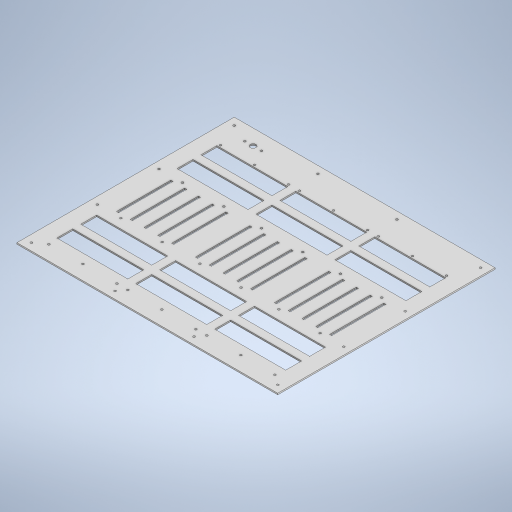
# Autodesk Inventor part: Pannello frontale
Saved by Autodesk Inventor 2023 (Build 270158000, 158)
## iProperties
Created: 2022-05-03
Part Number: Pannello frontale
Material: Generico
Document SubType Name: Sheet Metal
Designer: franc
Density: 1 g/cm^3
Sheet Metal Rule: Default_mm
Appearance: Default
Author: franc
Autodesk Inventor part; units mm, degrees
ref_plane "YZ Plane" through (0, 0, 0) normal (1, 0, 0) x (0, 1, 0)
ref_plane "XZ Plane" through (0, 0, 0) normal (0, 1, 0) x (-1, 0, 0)
ref_plane "XY Plane" through (0, 0, 0) normal (0, 0, 1) x (1, 0, 0)
sketch "Schizzo1" plane through (0, 0, 0) normal (0, 1, 0) x (-1, 0, 0)
  line L0 (270.7569, 212.2832) -> (267.7569, 212.2832)
  line L1 (270.7569, 137.2832) -> (267.7569, 137.2832)
  line L2 (270.7569, 137.2832) -> (270.7569, 212.2832)
  line L3 (267.7569, 137.2832) -> (267.7569, 212.2832)
  line L4 (289.7569, 212.2832) -> (286.7569, 212.2832)
  line L5 (289.7569, 137.2832) -> (286.7569, 137.2832)
  line L6 (289.7569, 137.2832) -> (289.7569, 212.2832)
  line L7 (286.7569, 137.2832) -> (286.7569, 212.2832)
  line L8 (308.7569, 212.2832) -> (305.7569, 212.2832)
  line L9 (308.7569, 137.2832) -> (305.7569, 137.2832)
  line L10 (308.7569, 137.2832) -> (308.7569, 212.2832)
  line L11 (305.7569, 137.2832) -> (305.7569, 212.2832)
  line L12 (327.7569, 212.2832) -> (324.7569, 212.2832)
  line L13 (327.7569, 137.2832) -> (324.7569, 137.2832)
  line L14 (327.7569, 137.2832) -> (327.7569, 212.2832)
  line L15 (324.7569, 137.2832) -> (324.7569, 212.2832)
  line L16 (346.7569, 212.2832) -> (343.7569, 212.2832)
  line L17 (346.7569, 137.2832) -> (343.7569, 137.2832)
  line L18 (346.7569, 137.2832) -> (346.7569, 212.2832)
  line L19 (343.7569, 137.2832) -> (343.7569, 212.2832)
  line L20 (71.7569, 137.2832) -> (68.7569, 137.2832)
  line L21 (71.7569, 137.2832) -> (71.7569, 212.2832)
  line L22 (68.7569, 137.2832) -> (68.7569, 212.2832)
  line L23 (343.7569, 137.2832) -> (346.7569, 137.2832)
  line L24 (90.7569, 137.2832) -> (87.7569, 137.2832)
  line L25 (90.7569, 137.2832) -> (90.7569, 212.2832)
  line L26 (87.7569, 137.2832) -> (87.7569, 212.2832)
  line L27 (109.7569, 212.2832) -> (106.7569, 212.2832)
  line L28 (109.7569, 137.2832) -> (106.7569, 137.2832)
  line L29 (109.7569, 137.2832) -> (109.7569, 212.2832)
  line L30 (106.7569, 137.2832) -> (106.7569, 212.2832)
  line L31 (128.7569, 212.2832) -> (125.7569, 212.2832)
  line L32 (128.7569, 137.2832) -> (125.7569, 137.2832)
  line L33 (128.7569, 137.2832) -> (128.7569, 212.2832)
  line L34 (125.7569, 137.2832) -> (125.7569, 212.2832)
  line L35 (138.2569, 263.2832) -> (40.2569, 263.2832)
  line L36 (90.7569, 212.2832) -> (87.7569, 212.2832)
  line L37 (40.2569, 263.2832) -> (40.2569, 285.2832)
  line L38 (40.2569, 285.2832) -> (138.2569, 285.2832)
  line L39 (138.2569, 285.2832) -> (138.2569, 263.2832)
  line L40 (378.2569, 18.2832) -> (18.2569, 18.2832)
  line L41 (18.2569, 18.2832) -> (18.2569, 318.2832)
  line L42 (18.2569, 318.2832) -> (378.2569, 318.2832)
  line L43 (378.2569, 318.2832) -> (378.2569, 18.2832)
  line L44 (161.7569, 212.2832) -> (158.7569, 212.2832)
  line L45 (161.7569, 137.2832) -> (158.7569, 137.2832)
  line L46 (161.7569, 137.2832) -> (161.7569, 212.2832)
  line L47 (158.7569, 137.2832) -> (158.7569, 212.2832)
  line L48 (180.7569, 212.2832) -> (177.7569, 212.2832)
  line L49 (180.7569, 137.2832) -> (177.7569, 137.2832)
  line L50 (180.7569, 137.2832) -> (180.7569, 212.2832)
  line L51 (177.7569, 137.2832) -> (177.7569, 212.2832)
  line L52 (199.7569, 212.2832) -> (196.7569, 212.2832)
  line L53 (199.7569, 137.2832) -> (196.7569, 137.2832)
  line L54 (199.7569, 137.2832) -> (199.7569, 212.2832)
  line L55 (196.7569, 137.2832) -> (196.7569, 212.2832)
  line L56 (218.7569, 212.2832) -> (215.7569, 212.2832)
  line L57 (218.7569, 137.2832) -> (215.7569, 137.2832)
  line L58 (218.7569, 137.2832) -> (218.7569, 212.2832)
  line L59 (215.7569, 137.2832) -> (215.7569, 212.2832)
  line L60 (237.7569, 212.2832) -> (234.7569, 212.2832)
  line L61 (237.7569, 137.2832) -> (234.7569, 137.2832)
  line L62 (237.7569, 137.2832) -> (237.7569, 212.2832)
  line L63 (234.7569, 137.2832) -> (234.7569, 212.2832)
  line L64 (52.7569, 212.2832) -> (49.7569, 212.2832)
  line L65 (52.7569, 137.2832) -> (49.7569, 137.2832)
  line L66 (52.7569, 137.2832) -> (52.7569, 212.2832)
  line L67 (49.7569, 137.2832) -> (49.7569, 212.2832)
  line L68 (71.7569, 212.2832) -> (68.7569, 212.2832)
  line L69 (149.2569, 263.2832) -> (149.2569, 285.2832)
  line L70 (138.2569, 230.2831) -> (40.2569, 230.2831)
  line L71 (40.2569, 230.2831) -> (40.2569, 252.2831)
  line L72 (40.2569, 252.2831) -> (138.2569, 252.2831)
  line L73 (138.2569, 252.2831) -> (138.2569, 230.2831)
  line L74 (138.2569, 97.2832) -> (40.2569, 97.2832)
  line L75 (40.2569, 97.2832) -> (40.2569, 119.2832)
  line L76 (40.2569, 119.2832) -> (138.2569, 119.2832)
  line L77 (138.2569, 119.2832) -> (138.2569, 97.2832)
  line L78 (138.2569, 64.2832) -> (40.2569, 64.2832)
  line L79 (40.2569, 64.2832) -> (40.2569, 86.2832)
  line L80 (40.2569, 86.2832) -> (138.2569, 86.2832)
  line L81 (138.2569, 86.2832) -> (138.2569, 64.2832)
  line L82 (247.2569, 263.2832) -> (149.2569, 263.2832)
  line L83 (149.2569, 285.2832) -> (247.2569, 285.2832)
  line L84 (247.2569, 285.2832) -> (247.2569, 263.2832)
  line L85 (247.2569, 230.2831) -> (149.2569, 230.2831)
  line L86 (149.2569, 230.2831) -> (149.2569, 252.2831)
  line L87 (149.2569, 252.2831) -> (247.2569, 252.2831)
  line L88 (247.2569, 252.2831) -> (247.2569, 230.2831)
  line L89 (247.2569, 97.2832) -> (149.2569, 97.2832)
  line L90 (149.2569, 97.2832) -> (149.2569, 119.2832)
  line L91 (149.2569, 119.2832) -> (247.2569, 119.2832)
  line L92 (247.2569, 119.2832) -> (247.2569, 97.2832)
  line L93 (247.2569, 64.2832) -> (149.2569, 64.2832)
  line L94 (149.2569, 64.2832) -> (149.2569, 86.2832)
  line L95 (149.2569, 86.2832) -> (247.2569, 86.2832)
  line L96 (247.2569, 86.2832) -> (247.2569, 64.2832)
  line L97 (356.2569, 263.2832) -> (258.2569, 263.2832)
  line L98 (258.2569, 263.2832) -> (258.2569, 285.2832)
  line L99 (258.2569, 285.2832) -> (356.2569, 285.2832)
  line L100 (356.2569, 285.2832) -> (356.2569, 263.2832)
  line L101 (356.2569, 230.2831) -> (258.2569, 230.2831)
  line L102 (258.2569, 230.2831) -> (258.2569, 252.2831)
  line L103 (258.2569, 252.2831) -> (356.2569, 252.2831)
  line L104 (356.2569, 252.2831) -> (356.2569, 230.2831)
  line L105 (356.2569, 97.2832) -> (258.2569, 97.2832)
  line L106 (258.2569, 97.2832) -> (258.2569, 119.2832)
  line L107 (258.2569, 119.2832) -> (356.2569, 119.2832)
  line L108 (356.2569, 119.2832) -> (356.2569, 97.2832)
  line L109 (356.2569, 64.2832) -> (258.2569, 64.2832)
  line L110 (258.2569, 64.2832) -> (258.2569, 86.2832)
  line L111 (258.2569, 86.2832) -> (356.2569, 86.2832)
  line L112 (356.2569, 86.2832) -> (356.2569, 64.2832)
  circle A0 centre (260.2569, 298.2832) radius 1.5
  circle A1 centre (245.2569, 61.2832) radius 1.5
  circle A2 centre (151.2569, 61.2832) radius 1.5
  circle A3 centre (245.2569, 298.2832) radius 1.5
  circle A4 centre (151.2569, 298.2832) radius 1.5
  circle A5 centre (136.2569, 61.2832) radius 1.5
  circle A6 centre (42.2569, 61.2832) radius 1.5
  circle A7 centre (136.2569, 298.2832) radius 1.5
  circle A8 centre (42.2569, 298.2832) radius 1.5
  circle A9 centre (136.2569, 61.2832) radius 1.5
  circle A10 centre (28.2569, 28.2832) radius 1.5
  circle A11 centre (28.2569, 308.2832) radius 1.5
  circle A12 centre (368.2569, 308.2832) radius 1.5
  circle A13 centre (342.2569, 39.7832) radius 1.5
  circle A14 centre (319.2569, 39.7832) radius 1.5
  circle A15 centre (330.7569, 39.7832) radius 4
  circle A16 centre (368.2569, 28.2832) radius 1.5
  circle A17 centre (252.7569, 308.2832) radius 1.5
  circle A18 centre (143.7569, 308.2832) radius 1.5
  circle A19 centre (252.7569, 28.2832) radius 1.5
  circle A20 centre (143.7569, 28.2832) radius 1.5
  circle A21 centre (354.2569, 61.2832) radius 1.5
  circle A22 centre (260.2569, 61.2832) radius 1.5
  circle A23 centre (354.2569, 298.2832) radius 1.5
  circle A24 centre (260.2569, 298.2832) radius 1.5
  circle A25 centre (245.2569, 61.2832) radius 1.5
  circle A26 centre (151.2569, 61.2832) radius 1.5
  circle A27 centre (245.2569, 298.2832) radius 1.5
  circle A28 centre (151.2569, 298.2832) radius 1.5
  circle A29 centre (136.2569, 61.2832) radius 1.5
  circle A30 centre (42.2569, 61.2832) radius 1.5
  circle A31 centre (136.2569, 298.2832) radius 1.5
  circle A32 centre (42.2569, 298.2832) radius 1.5
  circle A33 centre (354.2569, 61.2832) radius 1.5
  circle A34 centre (260.2569, 61.2832) radius 1.5
  circle A35 centre (354.2569, 298.2832) radius 1.5
  circle A36 centre (260.2569, 298.2832) radius 1.5
  circle A37 centre (245.2569, 61.2832) radius 1.5
  circle A38 centre (151.2569, 61.2832) radius 1.5
  circle A39 centre (245.2569, 298.2832) radius 1.5
  circle A40 centre (151.2569, 298.2832) radius 1.5
  circle A41 centre (136.2569, 61.2832) radius 1.5
  circle A42 centre (42.2569, 61.2832) radius 1.5
  circle A43 centre (136.2569, 298.2832) radius 1.5
  circle A44 centre (42.2569, 298.2832) radius 1.5
  circle A45 centre (28.2569, 28.2832) radius 1.5
  circle A46 centre (28.2569, 308.2832) radius 1.5
  circle A47 centre (368.2569, 308.2832) radius 1.5
  circle A48 centre (368.2569, 28.2832) radius 1.5
  circle A49 centre (252.7569, 308.2832) radius 1.5
  circle A50 centre (143.7569, 308.2832) radius 1.5
  circle A51 centre (252.7569, 28.2832) radius 1.5
  circle A52 centre (143.7569, 28.2832) radius 1.5
  circle A53 centre (136.2569, 61.2832) radius 1.5
  circle A54 centre (28.2569, 28.2832) radius 1.5
  circle A55 centre (28.2569, 308.2832) radius 1.5
  circle A56 centre (368.2569, 308.2832) radius 1.5
  circle A57 centre (368.2569, 28.2832) radius 1.5
  circle A58 centre (252.7569, 308.2832) radius 1.5
  circle A59 centre (143.7569, 308.2832) radius 1.5
  circle A60 centre (252.7569, 28.2832) radius 1.5
  circle A61 centre (143.7569, 28.2832) radius 1.5
  circle A62 centre (368.2569, 132.2832) radius 1.5
  circle A63 centre (368.2569, 217.2832) radius 1.5
  circle A64 centre (28.2569, 132.2832) radius 1.5
  circle A65 centre (28.2569, 217.2832) radius 1.5
  circle A66 centre (368.2569, 132.2832) radius 1.5
  circle A67 centre (368.2569, 217.2832) radius 1.5
  circle A68 centre (28.2569, 132.2832) radius 1.5
  circle A69 centre (28.2569, 217.2832) radius 1.5
  circle A70 centre (354.2569, 61.2832) radius 1.5
  circle A71 centre (260.2569, 61.2832) radius 1.5
  circle A72 centre (354.2569, 298.2832) radius 1.5
  circle A73 centre (260.2569, 298.2832) radius 1.5
  circle A74 centre (245.2569, 61.2832) radius 1.5
  circle A75 centre (151.2569, 61.2832) radius 1.5
  circle A76 centre (245.2569, 298.2832) radius 1.5
  circle A77 centre (151.2569, 298.2832) radius 1.5
  circle A78 centre (136.2569, 61.2832) radius 1.5
  circle A79 centre (42.2569, 61.2832) radius 1.5
  circle A80 centre (136.2569, 298.2832) radius 1.5
  circle A81 centre (42.2569, 298.2832) radius 1.5
  circle A82 centre (28.2569, 28.2832) radius 1.5
  circle A83 centre (28.2569, 308.2832) radius 1.5
  circle A84 centre (368.2569, 308.2832) radius 1.5
  circle A85 centre (368.2569, 28.2832) radius 1.5
  circle A86 centre (252.7569, 308.2832) radius 1.5
  circle A87 centre (143.7569, 308.2832) radius 1.5
  circle A88 centre (252.7569, 28.2832) radius 1.5
  circle A89 centre (143.7569, 28.2832) radius 1.5
  circle A90 centre (354.2569, 61.2832) radius 1.5
  circle A91 centre (260.2569, 61.2832) radius 1.5
  circle A92 centre (354.2569, 298.2832) radius 1.5
  circle A93 centre (260.2569, 298.2832) radius 1.5
  circle A94 centre (245.2569, 61.2832) radius 1.5
  circle A95 centre (151.2569, 61.2832) radius 1.5
  circle A96 centre (245.2569, 298.2832) radius 1.5
  circle A97 centre (151.2569, 298.2832) radius 1.5
  circle A98 centre (136.2569, 61.2832) radius 1.5
  circle A99 centre (42.2569, 61.2832) radius 1.5
  circle A100 centre (136.2569, 298.2832) radius 1.5
  circle A101 centre (42.2569, 298.2832) radius 1.5
  circle A102 centre (136.2569, 61.2832) radius 1.5
  circle A103 centre (28.2569, 28.2832) radius 1.5
  circle A104 centre (354.2569, 61.2832) radius 1.5
  circle A105 centre (368.2569, 308.2832) radius 1.5
  circle A106 centre (368.2569, 28.2832) radius 1.5
  circle A107 centre (252.7569, 308.2832) radius 1.5
  circle A108 centre (143.7569, 308.2832) radius 1.5
  circle A109 centre (252.7569, 28.2832) radius 1.5
  circle A110 centre (143.7569, 28.2832) radius 1.5
  circle A111 centre (354.2569, 61.2832) radius 1.5
  circle A112 centre (260.2569, 61.2832) radius 1.5
  circle A113 centre (354.2569, 298.2832) radius 1.5
  circle A114 centre (260.2569, 298.2832) radius 1.5
  circle A115 centre (245.2569, 61.2832) radius 1.5
  circle A116 centre (151.2569, 61.2832) radius 1.5
  circle A117 centre (245.2569, 298.2832) radius 1.5
  circle A118 centre (151.2569, 298.2832) radius 1.5
  circle A119 centre (136.2569, 61.2832) radius 1.5
  circle A120 centre (42.2569, 61.2832) radius 1.5
  circle A121 centre (136.2569, 298.2832) radius 1.5
  circle A122 centre (42.2569, 298.2832) radius 1.5
  circle A123 centre (368.2569, 132.2832) radius 1.5
  circle A124 centre (368.2569, 217.2832) radius 1.5
  circle A125 centre (28.2569, 132.2832) radius 1.5
  circle A126 centre (28.2569, 217.2832) radius 1.5
  circle A127 centre (307.2569, 61.2832) radius 1.5
  circle A128 centre (260.2569, 61.2832) radius 1.5
  circle A129 centre (354.2569, 298.2832) radius 1.5
  circle A130 centre (307.2569, 298.2832) radius 1.5
  circle A131 centre (260.2569, 298.2832) radius 1.5
  circle A132 centre (335.7569, 217.2832) radius 1.5
  circle A133 centre (278.7569, 217.2832) radius 1.5
  circle A134 centre (245.2569, 61.2832) radius 1.5
  circle A135 centre (198.2569, 61.2832) radius 1.5
  circle A136 centre (151.2569, 61.2832) radius 1.5
  circle A137 centre (245.2569, 298.2832) radius 1.5
  circle A138 centre (198.2569, 298.2832) radius 1.5
  circle A139 centre (151.2569, 298.2832) radius 1.5
  circle A140 centre (28.2569, 308.2832) radius 1.5
  circle A141 centre (136.2569, 61.2832) radius 1.5
  circle A142 centre (89.2569, 61.2832) radius 1.5
  circle A143 centre (136.2569, 298.2832) radius 1.5
  circle A144 centre (89.2569, 298.2832) radius 1.5
  circle A145 centre (42.2569, 298.2832) radius 1.5
  circle A146 centre (42.2569, 61.2832) radius 1.5
  circle A147 centre (226.7569, 217.2832) radius 1.5
  circle A148 centre (169.7569, 217.2832) radius 1.5
  circle A149 centre (117.7569, 217.2832) radius 1.5
  circle A150 centre (60.7569, 217.2832) radius 1.5
  circle A151 centre (335.7569, 132.2832) radius 1.5
  circle A152 centre (278.7569, 132.2832) radius 1.5
  circle A153 centre (226.7569, 132.2832) radius 1.5
  circle A154 centre (169.7569, 132.2832) radius 1.5
  circle A155 centre (117.7569, 132.2832) radius 1.5
  circle A156 centre (60.7569, 132.2832) radius 1.5
  circle A157 centre (28.2569, 28.2832) radius 1.5
  circle A158 centre (28.2569, 308.2832) radius 1.5
  circle A159 centre (368.2569, 308.2832) radius 1.5
  circle A160 centre (342.2569, 39.7832) radius 1.5
  circle A161 centre (319.2569, 39.7832) radius 1.5
  circle A162 centre (330.7569, 39.7832) radius 4
  circle A163 centre (368.2569, 28.2832) radius 1.5
  circle A164 centre (252.7569, 308.2832) radius 1.5
  circle A165 centre (143.7569, 308.2832) radius 1.5
  circle A166 centre (252.7569, 28.2832) radius 1.5
  circle A167 centre (143.7569, 28.2832) radius 1.5
  circle A168 centre (354.2569, 61.2832) radius 1.5
  circle A169 centre (260.2569, 61.2832) radius 1.5
  circle A170 centre (354.2569, 298.2832) radius 1.5
  point P0 (0, 0)
  constraints: 226 end point, 171 centre point
extrude "Estrusione1" add sketch "Schizzo1" along normal blind 2
equation "\"RaggioPiega\" = Spessore"
equation "\"LarghezzaScaricoPiega\" = Spessore"
equation "\"ProfonditàScaricoPiega\" = 0.5 * Spessore"
equation "\"DimensioniScaricoAngolo\" = 4 * Spessore"
equation "\"ResiduoMinimo\" = 2 * Spessore"
equation "\"RaggioTransizione\" = RaggioPiega"
equation "\"Dimensione_raggio_Jacobi\" = RaggioPiega"
equation "\"DimensioneGioco\" = Spessore"
equation "\"Spessore\" = 0.5"
